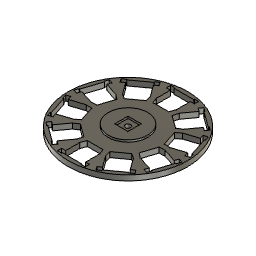
27.10_only_turel_cap (Autodesk Fusion 360 design; units mm, degrees)
Autodesk Fusion 360 part; units mm, degrees
(part 1 of 2)
sketch "Sketch1" plane through (0, 0, 0) normal (0, 0, 1) x (1, 0, 0)
  line L0 (0, -55) -> (0, -85)
  line L1 (0, -85) -> (18.6, -85)
  line L2 (18.6, -85) -> (18.6, -82.7)
  line L3 (18.6, -82.7) -> (13.6, -82.7)
  line L4 (0, -55) -> (5.5, -55)
  line L5 (0, -60) -> (12, -60) construction
  line L6 (5.5, -55) -> (12, -60)
  line L7 (12, -60) -> (13.6, -82.7)
  dimension "d1" = 30
  dimension "d3" = 18.6
  dimension "d4" = 2.3
  dimension "d5" = 5
  dimension "d6" = 5.5
  dimension "d7" = 12
  dimension "d8" = 5
  dimension "d20" = 85
  constraint vertical L0
  constraint coincident origin L0
  constraint perpendicular L0 L1
  constraint perpendicular L1 L2
  constraint perpendicular L2 L3
  constraint perpendicular L0 L4
  constraint coincident L0 L5.start
  constraint perpendicular L0 L5
  measures "d1" distance of L0.start L0.end
  measures "d3" distance of L0.end L1.end
  measures "d4" distance of L1.end L2.end
  measures "d5" distance of L2.end L3.end
  measures "d6" distance of L0.start L4.end
  measures "d7" distance of L5.start L5.end
  measures "d8" distance of L4 L5
  measures "d20" distance of origin L1
revolve "Revolve1" add sketch "Sketch1" angle 360 about axis through (0, -55, 0) along (0, -1, 0) makes body 1
sketch "Sketch2" plane through (0, 0, 0) normal (0, 0, 1) x (1, 0, 0)
  line L0 (-5.5, -55) -> (5.5, -55)
  line L1 (-18.6, -82.7) -> (-13.6, -82.7)
  line L2 (13.6, -82.7) -> (18.6, -82.7)
  line L3 (-18.6, -85) -> (18.6, -85)
  line L4 (-5.5, -55) -> (-12, -60)
  line L5 (5.5, -55) -> (12, -60)
  line L6 (-12, -60) -> (-13.6, -82.7)
  line L7 (12, -60) -> (13.6, -82.7)
  line L8 (-18.6, -82.7) -> (-18.6, -85)
  line L9 (18.6, -82.7) -> (18.6, -85)
  line L10 (0, -85) -> (0, -55) construction
  line L11 (-20.1, -85) -> (20.1, -85)
  line L12 (20.1, -85) -> (20.1, -81)
  line L13 (20.1, -81) -> (15.1, -81)
  line L14 (15.1, -81) -> (15.1, -58.2437)
  line L15 (-12, -60) -> (12, -60) construction
  line L16 (0, -55) -> (0, -50) construction
  line L17 (-12, -50) -> (12, -50)
  line L18 (15.1, -58.2437) -> (12, -50)
  line L19 (-15.1, -58.2437) -> (-12, -50)
  line L20 (-15.1, -81) -> (-15.1, -58.2437)
  line L21 (-20.1, -81) -> (-15.1, -81)
  line L22 (-20.1, -85) -> (-20.1, -81)
  dimension "d10" = 1.5
  dimension "d11" = 4
  dimension "d12" = 5
  dimension "d14" = 5
  constraint midpoint L3 L10.start
  constraint midpoint L0 L10.end
  constraint parallel L3 L11
  constraint midpoint L10.start L11
  constraint perpendicular L11 L12
  constraint perpendicular L12 L13
  constraint perpendicular L13 L14
  constraint equal L7 L14
  constraint coincident L4.end L6.start
  constraint coincident L5.end L7.start
  constraint perpendicular L0 L16
  constraint parallel L15 L17
  constraint midpoint L16.end L17
  constraint equal L15 L17
  constraint symmetric L10 L11.end L11.start
  constraint symmetric L10 L12.end L21.start
  constraint symmetric L10 L13.end L20.start
  constraint symmetric L10 L14.end L19.start
  constraint symmetric L10 L17.end L17.start
  measures "d10" distance of L3.end L11.end
  measures "d11" distance of L11.end L12.end
  measures "d12" distance of L12.end L13.end
  measures "d14" distance of L10.end L16.end
sketch "Sketch3" plane through (0, 0, 0) normal (0, 0, 1) x (1, 0, 0)
  line L0 (-12, -50) -> (12, -50)
  line L1 (15.1, -58.2437) -> (12, -50)
  line L2 (15.1, -81) -> (15.1, -58.2437)
  line L3 (-15.1, -81) -> (-15.1, -58.2437)
  line L4 (-15.1, -58.2437) -> (-12, -50)
  line L5 (20.1, -81) -> (15.1, -81)
  line L6 (-20.1, -85) -> (20.1, -85)
  line L7 (20.1, -85) -> (20.1, -81)
  line L8 (-20.1, -85) -> (-20.1, -81)
  line L9 (-20.1, -81) -> (-15.1, -81)
  circle A0 centre (0, 0) radius 91
  line L10 (-12, -50) -> (12, -50)
  line L11 (15.1, -58.2437) -> (15.1, -81)
  line L12 (20.1, -81) -> (20.1, -85)
  line L13 (20.1, -81) -> (15.1, -81)
  line L14 (15.1, -58.2437) -> (12, -50)
  line L15 (-12, -50) -> (-15.1, -58.2437)
  line L16 (-15.1, -58.2437) -> (-15.1, -81)
  line L17 (-15.1, -81) -> (-20.1, -81)
  line L18 (-20.1, -81) -> (-20.1, -85)
  line L19 (-20.1, -85) -> (20.1, -85)
  line L20 (19.6811, -47.5043) -> (39.0975, -33.3974)
  line L21 (46.4509, -38.2446) -> (39.0975, -33.3974)
  line L22 (46.4509, -38.2446) -> (59.8268, -56.6548)
  line L23 (63.8718, -53.7159) -> (59.8268, -56.6548)
  line L24 (63.8718, -53.7159) -> (66.223, -56.952)
  line L25 (33.7005, -80.5809) -> (66.223, -56.952)
  line L26 (31.3494, -77.3449) -> (33.7005, -80.5809)
  line L27 (35.3944, -74.4059) -> (31.3494, -77.3449)
  line L28 (22.0186, -55.9957) -> (35.3944, -74.4059)
  line L29 (19.6811, -47.5043) -> (22.0186, -55.9957)
  line L30 (43.8446, -26.8635) -> (51.261, -4.0382)
  line L31 (60.0592, -3.6373) -> (51.261, -4.0382)
  line L32 (60.0592, -3.6373) -> (81.7017, -10.6694)
  line L33 (83.2468, -5.9141) -> (81.7017, -10.6694)
  line L34 (83.2468, -5.9141) -> (87.051, -7.1502)
  line L35 (74.6286, -45.3827) -> (87.051, -7.1502)
  line L36 (70.8243, -44.1466) -> (74.6286, -45.3827)
  line L37 (72.3694, -39.3913) -> (70.8243, -44.1466)
  line L38 (50.7269, -32.3592) -> (72.3694, -39.3913)
  line L39 (43.8446, -26.8635) -> (50.7269, -32.3592)
  line L40 (51.261, 4.0382) -> (43.8446, 26.8635)
  line L41 (50.7269, 32.3592) -> (43.8446, 26.8635)
  line L42 (50.7269, 32.3592) -> (72.3694, 39.3913)
  line L43 (70.8243, 44.1466) -> (72.3694, 39.3913)
  line L44 (70.8243, 44.1466) -> (74.6286, 45.3827)
  line L45 (87.051, 7.1502) -> (74.6286, 45.3827)
  line L46 (83.2468, 5.9141) -> (87.051, 7.1502)
  line L47 (81.7017, 10.6694) -> (83.2468, 5.9141)
  line L48 (60.0592, 3.6373) -> (81.7017, 10.6694)
  line L49 (51.261, 4.0382) -> (60.0592, 3.6373)
  line L50 (39.0975, 33.3974) -> (19.6811, 47.5043)
  line L51 (22.0186, 55.9957) -> (19.6811, 47.5043)
  line L52 (22.0186, 55.9957) -> (35.3944, 74.4059)
  line L53 (31.3494, 77.3449) -> (35.3944, 74.4059)
  line L54 (31.3494, 77.3449) -> (33.7005, 80.5809)
  line L55 (66.223, 56.952) -> (33.7005, 80.5809)
  line L56 (63.8718, 53.7159) -> (66.223, 56.952)
  line L57 (59.8268, 56.6548) -> (63.8718, 53.7159)
  line L58 (46.4509, 38.2446) -> (59.8268, 56.6548)
  line L59 (39.0975, 33.3974) -> (46.4509, 38.2446)
  line L60 (12, 50) -> (-12, 50)
  line L61 (-15.1, 58.2437) -> (-12, 50)
  line L62 (-15.1, 58.2437) -> (-15.1, 81)
  line L63 (-20.1, 81) -> (-15.1, 81)
  line L64 (-20.1, 81) -> (-20.1, 85)
  line L65 (20.1, 85) -> (-20.1, 85)
  line L66 (20.1, 81) -> (20.1, 85)
  line L67 (15.1, 81) -> (20.1, 81)
  line L68 (15.1, 58.2437) -> (15.1, 81)
  line L69 (12, 50) -> (15.1, 58.2437)
  line L70 (-19.6811, 47.5043) -> (-39.0975, 33.3974)
  line L71 (-46.4509, 38.2446) -> (-39.0975, 33.3974)
  line L72 (-46.4509, 38.2446) -> (-59.8268, 56.6548)
  line L73 (-63.8718, 53.7159) -> (-59.8268, 56.6548)
  line L74 (-63.8718, 53.7159) -> (-66.223, 56.952)
  line L75 (-33.7005, 80.5809) -> (-66.223, 56.952)
  line L76 (-31.3494, 77.3449) -> (-33.7005, 80.5809)
  line L77 (-35.3944, 74.4059) -> (-31.3494, 77.3449)
  line L78 (-22.0186, 55.9957) -> (-35.3944, 74.4059)
  line L79 (-19.6811, 47.5043) -> (-22.0186, 55.9957)
  line L80 (-43.8446, 26.8635) -> (-51.261, 4.0382)
  line L81 (-60.0592, 3.6373) -> (-51.261, 4.0382)
  line L82 (-60.0592, 3.6373) -> (-81.7017, 10.6694)
  line L83 (-83.2468, 5.9141) -> (-81.7017, 10.6694)
  line L84 (-83.2468, 5.9141) -> (-87.051, 7.1502)
  line L85 (-74.6286, 45.3827) -> (-87.051, 7.1502)
  line L86 (-70.8243, 44.1466) -> (-74.6286, 45.3827)
  line L87 (-72.3694, 39.3913) -> (-70.8243, 44.1466)
  line L88 (-50.7269, 32.3592) -> (-72.3694, 39.3913)
  line L89 (-43.8446, 26.8635) -> (-50.7269, 32.3592)
  line L90 (-51.261, -4.0382) -> (-43.8446, -26.8635)
  line L91 (-50.7269, -32.3592) -> (-43.8446, -26.8635)
  line L92 (-50.7269, -32.3592) -> (-72.3694, -39.3913)
  line L93 (-70.8243, -44.1466) -> (-72.3694, -39.3913)
  line L94 (-70.8243, -44.1466) -> (-74.6286, -45.3827)
  line L95 (-87.051, -7.1502) -> (-74.6286, -45.3827)
  line L96 (-83.2468, -5.9141) -> (-87.051, -7.1502)
  line L97 (-81.7017, -10.6694) -> (-83.2468, -5.9141)
  line L98 (-60.0592, -3.6373) -> (-81.7017, -10.6694)
  line L99 (-51.261, -4.0382) -> (-60.0592, -3.6373)
  line L100 (-39.0975, -33.3974) -> (-19.6811, -47.5043)
  line L101 (-22.0186, -55.9957) -> (-19.6811, -47.5043)
  line L102 (-22.0186, -55.9957) -> (-35.3944, -74.4059)
  line L103 (-31.3494, -77.3449) -> (-35.3944, -74.4059)
  line L104 (-31.3494, -77.3449) -> (-33.7005, -80.5809)
  line L105 (-66.223, -56.952) -> (-33.7005, -80.5809)
  line L106 (-63.8718, -53.7159) -> (-66.223, -56.952)
  line L107 (-59.8268, -56.6548) -> (-63.8718, -53.7159)
  line L108 (-46.4509, -38.2446) -> (-59.8268, -56.6548)
  line L109 (-39.0975, -33.3974) -> (-46.4509, -38.2446)
  circle A1 centre (0, 0) radius 4.05
  dimension "d15" = 182
  dimension "d19" = 360
  dimension "d28" = 8.1
  constraint coincident A0.centre A1.centre
  constraint coincident L0.start L4.end
  constraint coincident L0.end L1.end
  constraint coincident L1.start L2.end
  constraint coincident L2.start L5.end
  constraint coincident L5.start L7.end
  constraint coincident L6.end L7.start
  constraint coincident L3.end L4.start
  constraint coincident L3.start L9.end
  constraint coincident L8.end L9.start
  constraint coincident L6.start L8.start
  measures "d15" diameter of A0
  measures "d28" diameter of A1
extrude "Extrude1" add sketch "Sketch3" along normal blind 8 separate body makes body 2
sketch "Sketch4" plane through (0, 0, 8) normal (0, 0, 1) x (-1, 0, 0)
  line L0 (43.8446, 26.8635) -> (50.7269, 32.3592)
  line L1 (50.7269, 32.3592) -> (72.3694, 39.3913)
  line L2 (72.3694, 39.3913) -> (70.8243, 44.1466)
  line L3 (70.8243, 44.1466) -> (74.6286, 45.3827)
  line L4 (74.6286, 45.3827) -> (87.051, 7.1502)
  line L5 (87.051, 7.1502) -> (83.2468, 5.9141)
  line L6 (83.2468, 5.9141) -> (81.7017, 10.6694)
  line L7 (81.7017, 10.6694) -> (60.0592, 3.6373)
  line L8 (60.0592, 3.6373) -> (51.261, 4.0382)
  line L9 (51.261, 4.0382) -> (43.8446, 26.8635)
  line L10 (19.6811, 47.5043) -> (22.0186, 55.9957)
  line L11 (22.0186, 55.9957) -> (35.3944, 74.4059)
  line L12 (35.3944, 74.4059) -> (31.3494, 77.3449)
  line L13 (31.3494, 77.3449) -> (33.7005, 80.5809)
  line L14 (33.7005, 80.5809) -> (66.223, 56.952)
  line L15 (66.223, 56.952) -> (63.8718, 53.7159)
  line L16 (63.8718, 53.7159) -> (59.8268, 56.6548)
  line L17 (59.8268, 56.6548) -> (46.4509, 38.2446)
  line L18 (46.4509, 38.2446) -> (39.0975, 33.3974)
  line L19 (39.0975, 33.3974) -> (19.6811, 47.5043)
  line L20 (51.261, -4.0382) -> (60.0592, -3.6373)
  line L21 (60.0592, -3.6373) -> (81.7017, -10.6694)
  line L22 (81.7017, -10.6694) -> (83.2468, -5.9141)
  line L23 (83.2468, -5.9141) -> (87.051, -7.1502)
  line L24 (87.051, -7.1502) -> (74.6286, -45.3827)
  line L25 (74.6286, -45.3827) -> (70.8243, -44.1466)
  line L26 (70.8243, -44.1466) -> (72.3694, -39.3913)
  line L27 (72.3694, -39.3913) -> (50.7269, -32.3592)
  line L28 (50.7269, -32.3592) -> (43.8446, -26.8635)
  line L29 (43.8446, -26.8635) -> (51.261, -4.0382)
  line L30 (12, -50) -> (15.1, -58.2437)
  line L31 (15.1, -58.2437) -> (15.1, -81)
  line L32 (15.1, -81) -> (20.1, -81)
  line L33 (20.1, -81) -> (20.1, -85)
  line L34 (20.1, -85) -> (-20.1, -85)
  line L35 (-20.1, -85) -> (-20.1, -81)
  line L36 (-20.1, -81) -> (-15.1, -81)
  line L37 (-15.1, -81) -> (-15.1, -58.2437)
  line L38 (-15.1, -58.2437) -> (-12, -50)
  line L39 (-12, -50) -> (12, -50)
  line L40 (-19.6811, -47.5043) -> (-22.0186, -55.9957)
  line L41 (-22.0186, -55.9957) -> (-35.3944, -74.4059)
  line L42 (-35.3944, -74.4059) -> (-31.3494, -77.3449)
  line L43 (-31.3494, -77.3449) -> (-33.7005, -80.5809)
  line L44 (-33.7005, -80.5809) -> (-66.223, -56.952)
  line L45 (-66.223, -56.952) -> (-63.8718, -53.7159)
  line L46 (-63.8718, -53.7159) -> (-59.8268, -56.6548)
  line L47 (-59.8268, -56.6548) -> (-46.4509, -38.2446)
  line L48 (-46.4509, -38.2446) -> (-39.0975, -33.3974)
  line L49 (-39.0975, -33.3974) -> (-19.6811, -47.5043)
  line L50 (-51.261, 4.0382) -> (-60.0592, 3.6373)
  line L51 (-60.0592, 3.6373) -> (-81.7017, 10.6694)
  line L52 (-81.7017, 10.6694) -> (-83.2468, 5.9141)
  line L53 (-83.2468, 5.9141) -> (-87.051, 7.1502)
  line L54 (-87.051, 7.1502) -> (-74.6286, 45.3827)
  line L55 (-74.6286, 45.3827) -> (-70.8243, 44.1466)
  line L56 (-70.8243, 44.1466) -> (-72.3694, 39.3913)
  line L57 (-72.3694, 39.3913) -> (-50.7269, 32.3592)
  line L58 (-50.7269, 32.3592) -> (-43.8446, 26.8635)
  line L59 (-43.8446, 26.8635) -> (-51.261, 4.0382)
  line L60 (15.1, 58.2437) -> (12, 50)
  line L61 (12, 50) -> (-12, 50)
  line L62 (-12, 50) -> (-15.1, 58.2437)
  line L63 (-15.1, 58.2437) -> (-15.1, 81)
  line L64 (-15.1, 81) -> (-20.1, 81)
  line L65 (-20.1, 81) -> (-20.1, 85)
  line L66 (-20.1, 85) -> (20.1, 85)
  line L67 (20.1, 85) -> (20.1, 81)
  line L68 (20.1, 81) -> (15.1, 81)
  line L69 (15.1, 81) -> (15.1, 58.2437)
  line L70 (-39.0975, 33.3974) -> (-46.4509, 38.2446)
  line L71 (-46.4509, 38.2446) -> (-59.8268, 56.6548)
  line L72 (-59.8268, 56.6548) -> (-63.8718, 53.7159)
  line L73 (-63.8718, 53.7159) -> (-66.223, 56.952)
  line L74 (-66.223, 56.952) -> (-33.7005, 80.5809)
  line L75 (-33.7005, 80.5809) -> (-31.3494, 77.3449)
  line L76 (-31.3494, 77.3449) -> (-35.3944, 74.4059)
  line L77 (-35.3944, 74.4059) -> (-22.0186, 55.9957)
  line L78 (-22.0186, 55.9957) -> (-19.6811, 47.5043)
  line L79 (-19.6811, 47.5043) -> (-39.0975, 33.3974)
  line L80 (39.0975, -33.3974) -> (46.4509, -38.2446)
  line L81 (46.4509, -38.2446) -> (59.8268, -56.6548)
  line L82 (59.8268, -56.6548) -> (63.8718, -53.7159)
  line L83 (63.8718, -53.7159) -> (66.223, -56.952)
  line L84 (66.223, -56.952) -> (33.7005, -80.5809)
  line L85 (33.7005, -80.5809) -> (31.3494, -77.3449)
  line L86 (31.3494, -77.3449) -> (35.3944, -74.4059)
  line L87 (35.3944, -74.4059) -> (22.0186, -55.9957)
  line L88 (22.0186, -55.9957) -> (19.6811, -47.5043)
  line L89 (19.6811, -47.5043) -> (39.0975, -33.3974)
  line L90 (-43.8446, -26.8635) -> (-50.7269, -32.3592)
  line L91 (-50.7269, -32.3592) -> (-72.3694, -39.3913)
  line L92 (-72.3694, -39.3913) -> (-70.8243, -44.1466)
  line L93 (-70.8243, -44.1466) -> (-74.6286, -45.3827)
  line L94 (-74.6286, -45.3827) -> (-87.051, -7.1502)
  line L95 (-87.051, -7.1502) -> (-83.2468, -5.9141)
  line L96 (-83.2468, -5.9141) -> (-81.7017, -10.6694)
  line L97 (-81.7017, -10.6694) -> (-60.0592, -3.6373)
  line L98 (-60.0592, -3.6373) -> (-51.261, -4.0382)
  line L99 (-51.261, -4.0382) -> (-43.8446, -26.8635)
  circle A0 centre (0, 0) radius 91
  line L100 (-20.1, 81) -> (-15.1, 81)
  line L101 (-20.1, 81) -> (-20.1, 85)
  line L102 (20.1, 85) -> (-20.1, 85)
  line L103 (20.1, 81) -> (20.1, 85)
  line L104 (15.1, 81) -> (20.1, 81)
  line L105 (-15.1, 81) -> (-20.1, 81)
  line L106 (-20.1, 85) -> (-20.1, 81)
  line L107 (-20.1, 85) -> (-14.95, 85)
  line L108 (-14.95, 85) -> (-14.95, 86.15)
  line L109 (-15.1, 81) -> (-15.1, 79.85)
  line L110 (-15.1, 79.85) -> (-21.25, 79.85)
  line L111 (-21.25, 79.85) -> (-21.25, 86.15)
  line L112 (-21.25, 86.15) -> (-14.95, 86.15)
  line L113 (0, 0) -> (0, 91) construction
  line L114 (15.1, 81) -> (15.1, 79.85)
  line L115 (15.1, 79.85) -> (21.25, 79.85)
  line L116 (21.25, 79.85) -> (21.25, 86.15)
  line L117 (21.25, 86.15) -> (14.95, 86.15)
  line L118 (14.95, 85) -> (14.95, 86.15)
  line L119 (20.1, 85) -> (14.95, 85)
  line L120 (20.1, 85) -> (20.1, 81)
  line L121 (15.1, 81) -> (20.1, 81)
  circle A1 centre (0, 0) radius 4.05
  dimension "d21" = 5.15
  dimension "d22" = 6.3
  dimension "d23" = 6.3
  constraint coincident L63.end L64.start
  constraint coincident L64.end L65.start
  constraint coincident L65.end L66.start
  constraint coincident L66 L107.end
  constraint perpendicular L65 L107
  constraint perpendicular L102 L108
  constraint coincident L63 L109.end
  constraint perpendicular L64 L109
  constraint perpendicular L63 L110
  constraint perpendicular L110 L111
  constraint perpendicular L108 L112
  constraint equal L108 L109
  constraint coincident A0.centre L113.start
  constraint coincident A0 L113.end
  constraint perpendicular L102 L113
  constraint symmetric L63.end L113 L68.end
  constraint symmetric L64.end L113 L67.end
  constraint symmetric L65.end L113 L66.end
  constraint symmetric L107.end L113 L118.start
  constraint symmetric L108.end L113 L117.end
  constraint symmetric L109.end L113 L114.end
  constraint symmetric L110.end L113 L115.end
  constraint symmetric L111.end L113 L116.end
  measures "d21" distance of L65.end L107.end
  measures "d22" distance of L108.end L111.end
  measures "d23" distance of L110.end L111.end
extrude "Extrude2" cut sketch "Sketch4" against normal blind 25 contours L66 L67 L68 L69 L102 L103 L104 L114 L115 L116 L117 L118 L119 L120 L121 | L63 L64 L65 L66 L100 L101 L102 L105 L106 L107 L108 L109 L110 L111 L112 bodies 2
pattern_circular "C-Pattern1" count 10 over 360 about axis through (0, 0, 1.75) along (0, 0, 1) of "Extrude2"
sketch "Sketch5" plane through (0, 0, 0) normal (0, 1, 0) x (1, 0, 0)
  line L0 (0, 0) -> (0, -592)
  dimension "d31" = 592
  constraint coincident L0.start origin
  constraint vertical L0
  measures "d31" distance of L0.start L0.end
ref_plane "WorkPlane1" through (0, 0, 296) normal (0, 0, 1) x (1, 0, 0)
sketch "Sketch6" plane through (0, 0, 8) normal (0, 0, 1) x (-1, 0, 0)
  line L0 (14.95, 85) -> (14.95, 86.15)
  line L1 (14.95, 86.15) -> (21.25, 86.15)
  line L2 (21.25, 86.15) -> (21.25, 79.85)
  line L3 (21.25, 79.85) -> (15.1, 79.85)
  line L4 (15.1, 79.85) -> (15.1, 58.2437)
  line L5 (15.1, 58.2437) -> (12, 50)
  line L6 (12, 50) -> (-12, 50)
  line L7 (-12, 50) -> (-15.1, 58.2437)
  line L8 (-15.1, 58.2437) -> (-15.1, 79.85)
  line L9 (-15.1, 79.85) -> (-21.25, 79.85)
  line L10 (-21.25, 79.85) -> (-21.25, 86.15)
  line L11 (-21.25, 86.15) -> (-14.95, 86.15)
  line L12 (-14.95, 86.15) -> (-14.95, 85)
  line L13 (-14.95, 85) -> (14.95, 85)
  circle A0 centre (0, 0) radius 4.05
  line L14 (85.4596, 12.0481) -> (86.5533, 12.4035)
  line L15 (86.5533, 12.4035) -> (88.5001, 6.4119)
  line L16 (88.5001, 6.4119) -> (82.5085, 4.4651)
  line L17 (82.5085, 4.4651) -> (80.608, 10.3141)
  line L18 (80.608, 10.3141) -> (60.0592, 3.6373)
  line L19 (60.0592, 3.6373) -> (51.261, 4.0382)
  line L20 (51.261, 4.0382) -> (43.8446, 26.8635)
  line L21 (43.8446, 26.8635) -> (50.7269, 32.3592)
  line L22 (50.7269, 32.3592) -> (71.2757, 39.036)
  line L23 (71.2757, 39.036) -> (69.3753, 44.885)
  line L24 (69.3753, 44.885) -> (75.3669, 46.8318)
  line L25 (75.3669, 46.8318) -> (77.3137, 40.8401)
  line L26 (77.3137, 40.8401) -> (76.22, 40.4847)
  line L27 (76.22, 40.4847) -> (85.4596, 12.0481)
  line L28 (62.0566, 59.9791) -> (62.7325, 60.9094)
  line L29 (62.7325, 60.9094) -> (67.8293, 57.2064)
  line L30 (67.8293, 57.2064) -> (64.1263, 52.1096)
  line L31 (64.1263, 52.1096) -> (59.1508, 55.7244)
  line L32 (59.1508, 55.7244) -> (46.4509, 38.2446)
  line L33 (46.4509, 38.2446) -> (39.0975, 33.3974)
  line L34 (39.0975, 33.3974) -> (19.6811, 47.5043)
  line L35 (19.6811, 47.5043) -> (22.0186, 55.9957)
  line L36 (22.0186, 55.9957) -> (34.7185, 73.4756)
  line L37 (34.7185, 73.4756) -> (29.743, 77.0904)
  line L38 (29.743, 77.0904) -> (33.4461, 82.1873)
  line L39 (33.4461, 82.1873) -> (38.5429, 78.4842)
  line L40 (38.5429, 78.4842) -> (37.8669, 77.5538)
  line L41 (37.8669, 77.5538) -> (62.0566, 59.9791)
  line L42 (-14.95, -85) -> (-14.95, -86.15)
  line L43 (-14.95, -86.15) -> (-21.25, -86.15)
  line L44 (-21.25, -86.15) -> (-21.25, -79.85)
  line L45 (-21.25, -79.85) -> (-15.1, -79.85)
  line L46 (-15.1, -79.85) -> (-15.1, -58.2437)
  line L47 (-15.1, -58.2437) -> (-12, -50)
  line L48 (-12, -50) -> (12, -50)
  line L49 (12, -50) -> (15.1, -58.2437)
  line L50 (15.1, -58.2437) -> (15.1, -79.85)
  line L51 (15.1, -79.85) -> (21.25, -79.85)
  line L52 (21.25, -79.85) -> (21.25, -86.15)
  line L53 (21.25, -86.15) -> (14.95, -86.15)
  line L54 (14.95, -86.15) -> (14.95, -85)
  line L55 (14.95, -85) -> (-14.95, -85)
  line L56 (37.8669, -77.5538) -> (38.5429, -78.4842)
  line L57 (38.5429, -78.4842) -> (33.4461, -82.1873)
  line L58 (33.4461, -82.1873) -> (29.743, -77.0904)
  line L59 (29.743, -77.0904) -> (34.7185, -73.4756)
  line L60 (34.7185, -73.4756) -> (22.0186, -55.9957)
  line L61 (22.0186, -55.9957) -> (19.6811, -47.5043)
  line L62 (19.6811, -47.5043) -> (39.0975, -33.3974)
  line L63 (39.0975, -33.3974) -> (46.4509, -38.2446)
  line L64 (46.4509, -38.2446) -> (59.1508, -55.7244)
  line L65 (59.1508, -55.7244) -> (64.1263, -52.1096)
  line L66 (64.1263, -52.1096) -> (67.8293, -57.2064)
  line L67 (67.8293, -57.2064) -> (62.7325, -60.9094)
  line L68 (62.7325, -60.9094) -> (62.0566, -59.9791)
  line L69 (62.0566, -59.9791) -> (37.8669, -77.5538)
  line L70 (-85.4596, -12.0481) -> (-86.5533, -12.4035)
  line L71 (-86.5533, -12.4035) -> (-88.5001, -6.4119)
  line L72 (-88.5001, -6.4119) -> (-82.5085, -4.4651)
  line L73 (-82.5085, -4.4651) -> (-80.608, -10.3141)
  line L74 (-80.608, -10.3141) -> (-60.0592, -3.6373)
  line L75 (-60.0592, -3.6373) -> (-51.261, -4.0382)
  line L76 (-51.261, -4.0382) -> (-43.8446, -26.8635)
  line L77 (-43.8446, -26.8635) -> (-50.7269, -32.3592)
  line L78 (-50.7269, -32.3592) -> (-71.2757, -39.036)
  line L79 (-71.2757, -39.036) -> (-69.3753, -44.885)
  line L80 (-69.3753, -44.885) -> (-75.3669, -46.8318)
  line L81 (-75.3669, -46.8318) -> (-77.3137, -40.8401)
  line L82 (-77.3137, -40.8401) -> (-76.22, -40.4847)
  line L83 (-76.22, -40.4847) -> (-85.4596, -12.0481)
  line L84 (-76.22, 40.4847) -> (-77.3137, 40.8401)
  line L85 (-77.3137, 40.8401) -> (-75.3669, 46.8318)
  line L86 (-75.3669, 46.8318) -> (-69.3753, 44.885)
  line L87 (-69.3753, 44.885) -> (-71.2757, 39.036)
  line L88 (-71.2757, 39.036) -> (-50.7269, 32.3592)
  line L89 (-50.7269, 32.3592) -> (-43.8446, 26.8635)
  line L90 (-43.8446, 26.8635) -> (-51.261, 4.0382)
  line L91 (-51.261, 4.0382) -> (-60.0592, 3.6373)
  line L92 (-60.0592, 3.6373) -> (-80.608, 10.3141)
  line L93 (-80.608, 10.3141) -> (-82.5085, 4.4651)
  line L94 (-82.5085, 4.4651) -> (-88.5001, 6.4119)
  line L95 (-88.5001, 6.4119) -> (-86.5533, 12.4035)
  line L96 (-86.5533, 12.4035) -> (-85.4596, 12.0481)
  line L97 (-85.4596, 12.0481) -> (-76.22, 40.4847)
  line L98 (-62.0566, -59.9791) -> (-62.7325, -60.9094)
  line L99 (-62.7325, -60.9094) -> (-67.8293, -57.2064)
  line L100 (-67.8293, -57.2064) -> (-64.1263, -52.1096)
  line L101 (-64.1263, -52.1096) -> (-59.1508, -55.7244)
  line L102 (-59.1508, -55.7244) -> (-46.4509, -38.2446)
  line L103 (-46.4509, -38.2446) -> (-39.0975, -33.3974)
  line L104 (-39.0975, -33.3974) -> (-19.6811, -47.5043)
  line L105 (-19.6811, -47.5043) -> (-22.0186, -55.9957)
  line L106 (-22.0186, -55.9957) -> (-34.7185, -73.4756)
  line L107 (-34.7185, -73.4756) -> (-29.743, -77.0904)
  line L108 (-29.743, -77.0904) -> (-33.4461, -82.1873)
  line L109 (-33.4461, -82.1873) -> (-38.5429, -78.4842)
  line L110 (-38.5429, -78.4842) -> (-37.8669, -77.5538)
  line L111 (-37.8669, -77.5538) -> (-62.0566, -59.9791)
  line L112 (76.22, -40.4847) -> (77.3137, -40.8401)
  line L113 (77.3137, -40.8401) -> (75.3669, -46.8318)
  line L114 (75.3669, -46.8318) -> (69.3753, -44.885)
  line L115 (69.3753, -44.885) -> (71.2757, -39.036)
  line L116 (71.2757, -39.036) -> (50.7269, -32.3592)
  line L117 (50.7269, -32.3592) -> (43.8446, -26.8635)
  line L118 (43.8446, -26.8635) -> (51.261, -4.0382)
  line L119 (51.261, -4.0382) -> (60.0592, -3.6373)
  line L120 (60.0592, -3.6373) -> (80.608, -10.3141)
  line L121 (80.608, -10.3141) -> (82.5085, -4.4651)
  line L122 (82.5085, -4.4651) -> (88.5001, -6.4119)
  line L123 (88.5001, -6.4119) -> (86.5533, -12.4035)
  line L124 (86.5533, -12.4035) -> (85.4596, -12.0481)
  line L125 (85.4596, -12.0481) -> (76.22, -40.4847)
  line L126 (-37.8669, 77.5538) -> (-38.5429, 78.4842)
  line L127 (-38.5429, 78.4842) -> (-33.4461, 82.1873)
  line L128 (-33.4461, 82.1873) -> (-29.743, 77.0904)
  line L129 (-29.743, 77.0904) -> (-34.7185, 73.4756)
  line L130 (-34.7185, 73.4756) -> (-22.0186, 55.9957)
  line L131 (-22.0186, 55.9957) -> (-19.6811, 47.5043)
  line L132 (-19.6811, 47.5043) -> (-39.0975, 33.3974)
  line L133 (-39.0975, 33.3974) -> (-46.4509, 38.2446)
  line L134 (-46.4509, 38.2446) -> (-59.1508, 55.7244)
  line L135 (-59.1508, 55.7244) -> (-64.1263, 52.1096)
  line L136 (-64.1263, 52.1096) -> (-67.8293, 57.2064)
  line L137 (-67.8293, 57.2064) -> (-62.7325, 60.9094)
  line L138 (-62.7325, 60.9094) -> (-62.0566, 59.9791)
  line L139 (-62.0566, 59.9791) -> (-37.8669, 77.5538)
  circle A1 centre (0, 0) radius 91
  line L140 (10.075, -10.075) -> (-10.075, -10.075)
  line L141 (-10.075, -10.075) -> (-10.075, 10.075)
  line L142 (-10.075, 10.075) -> (10.075, 10.075)
  line L143 (10.075, 10.075) -> (10.075, -10.075)
  line L144 (10.075, -10.075) -> (-10.075, 10.075) construction
  circle A2 centre (0, 0) radius 30
  line L145 (20.1, 85) -> (-20.1, 85)
  line L146 (-20.1, 81) -> (-20.1, 85)
  line L147 (-20.1, 81) -> (-15.1, 81)
  line L148 (-15.1, 58.2437) -> (-15.1, 81)
  line L149 (15.1, 58.2437) -> (15.1, 81)
  line L150 (15.1, 81) -> (20.1, 81)
  line L151 (20.1, 81) -> (20.1, 85)
  line L152 (10.3486, 85) -> (-10.3486, 85)
  arc A3 (10.3486, 85) -> (-15.1, 81) centre (0, 67.8855) ccw
  line L153 (-41.5895, 74.8492) -> (-58.334, 62.6837)
  arc A4 (-41.5895, 74.8492) -> (-59.8268, 56.6548) centre (-39.9021, 54.9205) ccw
  line L154 (-77.6419, 36.1086) -> (-84.0377, 16.4243)
  arc A5 (-77.6419, 36.1086) -> (-81.7017, 10.6694) centre (-64.563, 20.9778) ccw
  line L155 (-84.0377, -16.4243) -> (-77.6419, -36.1086)
  arc A6 (-84.0377, -16.4243) -> (-72.3694, -39.3913) centre (-64.563, -20.9778) ccw
  line L156 (-58.334, -62.6837) -> (-41.5895, -74.8492)
  arc A7 (-58.334, -62.6837) -> (-35.3944, -74.4059) centre (-39.9021, -54.9205) ccw
  line L157 (-10.3486, -85) -> (10.3486, -85)
  arc A8 (-10.3486, -85) -> (15.1, -81) centre (0, -67.8855) ccw
  line L158 (41.5895, -74.8492) -> (58.334, -62.6837)
  arc A9 (41.5895, -74.8492) -> (59.8268, -56.6548) centre (39.9021, -54.9205) ccw
  line L159 (77.6419, -36.1086) -> (84.0377, -16.4243)
  arc A10 (77.6419, -36.1086) -> (81.7017, -10.6694) centre (64.563, -20.9778) ccw
  line L160 (84.0377, 16.4243) -> (77.6419, 36.1086)
  arc A11 (84.0377, 16.4243) -> (72.3694, 39.3913) centre (64.563, 20.9778) ccw
  line L161 (58.334, 62.6837) -> (41.5895, 74.8492)
  arc A12 (58.334, 62.6837) -> (35.3944, 74.4059) centre (39.9021, 54.9205) ccw
  arc A13 (-29.743, -77.0904) -> (-21.25, -79.85) centre (-19.1862, -59.0492) ccw
  line L162 (0, 0) -> (-1.4578, -3.7785)
  line L163 (-10.7987, -27.9891) -> (-29.743, -77.0904)
  line L164 (0, 0) -> (-1.0416, -3.9138)
  line L165 (-7.7152, -28.991) -> (-21.25, -79.85)
  line L166 (7.7152, -28.991) -> (21.25, -79.85)
  arc A14 (21.25, -79.85) -> (29.743, -77.0904) centre (19.1862, -59.0492) ccw
  line L167 (10.7987, -27.9891) -> (29.743, -77.0904)
  line L168 (23.2822, -18.9193) -> (64.1263, -52.1096)
  arc A15 (64.1263, -52.1096) -> (69.3753, -44.885) centre (50.2302, -36.4944) ccw
  line L169 (25.1879, -16.2963) -> (69.3753, -44.885)
  line L170 (29.9562, -1.6211) -> (82.5085, -4.4651)
  arc A16 (82.5085, -4.4651) -> (82.5085, 4.4651) centre (62.088, 0) ccw
  line L171 (29.9562, 1.6211) -> (82.5085, 4.4651)
  line L172 (25.1879, 16.2963) -> (69.3753, 44.885)
  arc A17 (69.3753, 44.885) -> (64.1263, 52.1096) centre (50.2302, 36.4944) ccw
  line L173 (23.2822, 18.9193) -> (64.1263, 52.1096)
  line L174 (10.7987, 27.9891) -> (29.743, 77.0904)
  arc A18 (29.743, 77.0904) -> (21.25, 79.85) centre (19.1862, 59.0492) ccw
  line L175 (7.7152, 28.991) -> (21.25, 79.85)
  line L176 (-7.7152, 28.991) -> (-21.25, 79.85)
  arc A19 (-21.25, 79.85) -> (-29.743, 77.0904) centre (-19.1862, 59.0492) ccw
  line L177 (-10.7987, 27.9891) -> (-29.743, 77.0904)
  line L178 (-23.2822, 18.9193) -> (-64.1263, 52.1096)
  arc A20 (-64.1263, 52.1096) -> (-69.3753, 44.885) centre (-50.2302, 36.4944) ccw
  line L179 (-25.1879, 16.2963) -> (-69.3753, 44.885)
  line L180 (-29.9562, 1.6211) -> (-82.5085, 4.4651)
  arc A21 (-82.5085, 4.4651) -> (-82.5085, -4.4651) centre (-62.088, 0) ccw
  line L181 (-29.9562, -1.6211) -> (-82.5085, -4.4651)
  line L182 (-25.1879, -16.2963) -> (-69.3753, -44.885)
  arc A22 (-69.3753, -44.885) -> (-64.1263, -52.1096) centre (-50.2302, -36.4944) ccw
  line L183 (-23.2822, -18.9193) -> (-64.1263, -52.1096)
  line L184 (0, 0) -> (0, 91) construction
  dimension "d35" = 20.15
  dimension "d36" = 60
  dimension "d44" = 40
  dimension "d47" = 360
  dimension "d93" = 62.088
  dimension "d95" = 360
  constraint horizontal L140
  constraint vertical L141
  constraint horizontal L142
  constraint vertical L143
  constraint equal L140 L141
  constraint midpoint A0.centre L144
  constraint coincident A0.centre A1.centre
  constraint coincident L13 L152.start
  constraint coincident L145 L152.end
  constraint coincident L152.end A3
  constraint coincident L107.end L108.start
  constraint coincident L44.end L45.start
  constraint coincident A2 L163.start
  constraint collinear L162 L163
  constraint coincident A2 L165.start
  constraint collinear L164 L165
  constraint coincident A0 L162.end
  constraint coincident A0 L164.end
  constraint coincident A1 L184.end
  constraint perpendicular L145 L184
  constraint coincident L149.end A3
  measures "d35" distance of L140.start L140.end
  measures "d36" diameter of A2
  measures "d44" diameter of A3
  measures "d93" distance of A0.centre A13.centre
extrude "Extrude3" add sketch "Sketch6" along normal blind 3 contours A2 bodies 2
extrude "Extrude4" [rolled back] along distance -1 taper angle 0
sketch "Sketch7" plane through (0, 0, 0) normal (0, 0, -1) x (1, 0, 0)
  circle A0 centre (0, 0) radius 4.05
  line L0 (-50.7269, 32.3592) -> (-43.8446, 26.8635)
  line L1 (-43.8446, 26.8635) -> (-51.261, 4.0382)
  line L2 (-51.261, 4.0382) -> (-60.0592, 3.6373)
  line L3 (-60.0592, 3.6373) -> (-81.7017, 10.6694)
  line L4 (-81.7017, 10.6694) -> (-83.2468, 5.9141)
  line L5 (-83.2468, 5.9141) -> (-87.051, 7.1502)
  line L6 (-87.051, 7.1502) -> (-74.6286, 45.3827)
  line L7 (-74.6286, 45.3827) -> (-70.8243, 44.1466)
  line L8 (-70.8243, 44.1466) -> (-72.3694, 39.3913)
  line L9 (-72.3694, 39.3913) -> (-50.7269, 32.3592)
  line L10 (-22.0186, 55.9957) -> (-19.6811, 47.5043)
  line L11 (-19.6811, 47.5043) -> (-39.0975, 33.3974)
  line L12 (-39.0975, 33.3974) -> (-46.4509, 38.2446)
  line L13 (-46.4509, 38.2446) -> (-59.8268, 56.6548)
  line L14 (-59.8268, 56.6548) -> (-63.8718, 53.7159)
  line L15 (-63.8718, 53.7159) -> (-66.223, 56.952)
  line L16 (-66.223, 56.952) -> (-33.7005, 80.5809)
  line L17 (-33.7005, 80.5809) -> (-31.3494, 77.3449)
  line L18 (-31.3494, 77.3449) -> (-35.3944, 74.4059)
  line L19 (-35.3944, 74.4059) -> (-22.0186, 55.9957)
  line L20 (-15.1, -58.2437) -> (-12, -50)
  line L21 (-12, -50) -> (12, -50)
  line L22 (12, -50) -> (15.1, -58.2437)
  line L23 (15.1, -58.2437) -> (15.1, -81)
  line L24 (15.1, -81) -> (20.1, -81)
  line L25 (20.1, -81) -> (20.1, -85)
  line L26 (20.1, -85) -> (-20.1, -85)
  line L27 (-20.1, -85) -> (-20.1, -81)
  line L28 (-20.1, -81) -> (-15.1, -81)
  line L29 (-15.1, -81) -> (-15.1, -58.2437)
  line L30 (-46.4509, -38.2446) -> (-39.0975, -33.3974)
  line L31 (-39.0975, -33.3974) -> (-19.6811, -47.5043)
  line L32 (-19.6811, -47.5043) -> (-22.0186, -55.9957)
  line L33 (-22.0186, -55.9957) -> (-35.3944, -74.4059)
  line L34 (-35.3944, -74.4059) -> (-31.3494, -77.3449)
  line L35 (-31.3494, -77.3449) -> (-33.7005, -80.5809)
  line L36 (-33.7005, -80.5809) -> (-66.223, -56.952)
  line L37 (-66.223, -56.952) -> (-63.8718, -53.7159)
  line L38 (-63.8718, -53.7159) -> (-59.8268, -56.6548)
  line L39 (-59.8268, -56.6548) -> (-46.4509, -38.2446)
  line L40 (50.7269, -32.3592) -> (43.8446, -26.8635)
  line L41 (43.8446, -26.8635) -> (51.261, -4.0382)
  line L42 (51.261, -4.0382) -> (60.0592, -3.6373)
  line L43 (60.0592, -3.6373) -> (81.7017, -10.6694)
  line L44 (81.7017, -10.6694) -> (83.2468, -5.9141)
  line L45 (83.2468, -5.9141) -> (87.051, -7.1502)
  line L46 (87.051, -7.1502) -> (74.6286, -45.3827)
  line L47 (74.6286, -45.3827) -> (70.8243, -44.1466)
  line L48 (70.8243, -44.1466) -> (72.3694, -39.3913)
  line L49 (72.3694, -39.3913) -> (50.7269, -32.3592)
  line L50 (60.0592, 3.6373) -> (51.261, 4.0382)
  line L51 (51.261, 4.0382) -> (43.8446, 26.8635)
  line L52 (43.8446, 26.8635) -> (50.7269, 32.3592)
  line L53 (50.7269, 32.3592) -> (72.3694, 39.3913)
  line L54 (72.3694, 39.3913) -> (70.8243, 44.1466)
  line L55 (70.8243, 44.1466) -> (74.6286, 45.3827)
  line L56 (74.6286, 45.3827) -> (87.051, 7.1502)
  line L57 (87.051, 7.1502) -> (83.2468, 5.9141)
  line L58 (83.2468, 5.9141) -> (81.7017, 10.6694)
  line L59 (81.7017, 10.6694) -> (60.0592, 3.6373)
  line L60 (22.0186, -55.9957) -> (19.6811, -47.5043)
  line L61 (19.6811, -47.5043) -> (39.0975, -33.3974)
  line L62 (39.0975, -33.3974) -> (46.4509, -38.2446)
  line L63 (46.4509, -38.2446) -> (59.8268, -56.6548)
  line L64 (59.8268, -56.6548) -> (63.8718, -53.7159)
  line L65 (63.8718, -53.7159) -> (66.223, -56.952)
  line L66 (66.223, -56.952) -> (33.7005, -80.5809)
  line L67 (33.7005, -80.5809) -> (31.3494, -77.3449)
  line L68 (31.3494, -77.3449) -> (35.3944, -74.4059)
  line L69 (35.3944, -74.4059) -> (22.0186, -55.9957)
  line L70 (-12, 50) -> (-15.1, 58.2437)
  line L71 (-15.1, 58.2437) -> (-15.1, 81)
  line L72 (-15.1, 81) -> (-20.1, 81)
  line L73 (-20.1, 81) -> (-20.1, 85)
  line L74 (-20.1, 85) -> (20.1, 85)
  line L75 (20.1, 85) -> (20.1, 81)
  line L76 (20.1, 81) -> (15.1, 81)
  line L77 (15.1, 81) -> (15.1, 58.2437)
  line L78 (15.1, 58.2437) -> (12, 50)
  line L79 (12, 50) -> (-12, 50)
  line L80 (-60.0592, -3.6373) -> (-51.261, -4.0382)
  line L81 (-51.261, -4.0382) -> (-43.8446, -26.8635)
  line L82 (-43.8446, -26.8635) -> (-50.7269, -32.3592)
  line L83 (-50.7269, -32.3592) -> (-72.3694, -39.3913)
  line L84 (-72.3694, -39.3913) -> (-70.8243, -44.1466)
  line L85 (-70.8243, -44.1466) -> (-74.6286, -45.3827)
  line L86 (-74.6286, -45.3827) -> (-87.051, -7.1502)
  line L87 (-87.051, -7.1502) -> (-83.2468, -5.9141)
  line L88 (-83.2468, -5.9141) -> (-81.7017, -10.6694)
  line L89 (-81.7017, -10.6694) -> (-60.0592, -3.6373)
  line L90 (46.4509, 38.2446) -> (39.0975, 33.3974)
  line L91 (39.0975, 33.3974) -> (19.6811, 47.5043)
  line L92 (19.6811, 47.5043) -> (22.0186, 55.9957)
  line L93 (22.0186, 55.9957) -> (35.3944, 74.4059)
  line L94 (35.3944, 74.4059) -> (31.3494, 77.3449)
  line L95 (31.3494, 77.3449) -> (33.7005, 80.5809)
  line L96 (33.7005, 80.5809) -> (66.223, 56.952)
  line L97 (66.223, 56.952) -> (63.8718, 53.7159)
  line L98 (63.8718, 53.7159) -> (59.8268, 56.6548)
  line L99 (59.8268, 56.6548) -> (46.4509, 38.2446)
  circle A1 centre (0, 0) radius 91
  circle A2 centre (0, 0) radius 26.55
  line L100 (-15.1, 58.2437) -> (-15.1, 81)
  line L101 (-12, 50) -> (-15.1, 58.2437)
  line L102 (-12, 50) -> (12, 50)
  line L103 (15.1, 58.2437) -> (12, 50)
  line L104 (15.1, 58.2437) -> (15.1, 81)
  line L105 (20.1, 81) -> (15.1, 81)
  line L106 (20.1, 81) -> (20.1, 85)
  line L107 (-20.1, 85) -> (20.1, 85)
  line L108 (-20.1, 81) -> (-20.1, 85)
  line L109 (-15.1, 81) -> (-20.1, 81)
  arc A3 (15.1, 81) -> (-10.3486, 85) centre (0, 67.8855) ccw
  dimension "d41" = 53.1
  constraint concentric A0 A2
  measures "d41" diameter of A2
extrude "Extrude5" [rolled back] along distance -3.5 taper angle 0
extrude "Extrude6" [rolled back] taper angle 0
ref_plane "WorkPlane6" through (0, 0, -10) normal (0, 0, 1) x (1, 0, 0)
sketch "Sketch10" plane through (0, 0, -10) normal (0, 0, 1) x (1, 0, 0)
  arc A0 (41.5895, -74.8492) -> (58.334, -62.6837) centre (39.9021, -54.9205) ccw
  arc A1 (58.334, 62.6837) -> (41.5895, 74.8492) centre (39.9021, 54.9205) ccw
  arc A2 (-77.6419, 36.1086) -> (-84.0377, 16.4243) centre (-64.563, 20.9778) ccw
  arc A3 (10.3486, 85) -> (-10.3486, 85) centre (0, 67.8855) ccw
  arc A4 (-10.3486, -85) -> (10.3486, -85) centre (0, -67.8855) ccw
  arc A5 (77.6419, -36.1086) -> (84.0377, -16.4243) centre (64.563, -20.9778) ccw
  arc A6 (-41.5895, 74.8492) -> (-58.334, 62.6837) centre (-39.9021, 54.9205) ccw
  arc A7 (-84.0377, -16.4243) -> (-77.6419, -36.1086) centre (-64.563, -20.9778) ccw
  arc A8 (84.0377, 16.4243) -> (77.6419, 36.1086) centre (64.563, 20.9778) ccw
  arc A9 (-58.334, -62.6837) -> (-41.5895, -74.8492) centre (-39.9021, -54.9205) ccw
  line L0 (66.223, -56.952) -> (58.334, -62.6837)
  line L1 (33.7005, 80.5809) -> (41.5895, 74.8492)
  line L2 (-87.051, 7.1502) -> (-84.0377, 16.4243)
  line L3 (-20.1, 85) -> (-10.3486, 85)
  line L4 (20.1, -85) -> (10.3486, -85)
  line L5 (87.051, -7.1502) -> (84.0377, -16.4243)
  line L6 (-66.223, 56.952) -> (-58.334, 62.6837)
  line L7 (-74.6286, -45.3827) -> (-77.6419, -36.1086)
  line L8 (74.6286, 45.3827) -> (77.6419, 36.1086)
  line L9 (-70.8243, -44.1466) -> (-74.6286, -45.3827)
  line L10 (-72.3694, -39.3913) -> (-70.8243, -44.1466)
  line L11 (-50.7269, -32.3592) -> (-72.3694, -39.3913)
  line L12 (-43.8446, -26.8635) -> (-50.7269, -32.3592)
  line L13 (-51.261, -4.0382) -> (-43.8446, -26.8635)
  line L14 (-60.0592, -3.6373) -> (-51.261, -4.0382)
  line L15 (-81.7017, -10.6694) -> (-60.0592, -3.6373)
  line L16 (-83.2468, -5.9141) -> (-81.7017, -10.6694)
  line L17 (-87.051, -7.1502) -> (-83.2468, -5.9141)
  line L18 (-84.0377, -16.4243) -> (-87.051, -7.1502)
  line L19 (-33.7005, -80.5809) -> (-41.5895, -74.8492)
  line L20 (-31.3494, -77.3449) -> (-33.7005, -80.5809)
  line L21 (-35.3944, -74.4059) -> (-31.3494, -77.3449)
  line L22 (-22.0186, -55.9957) -> (-35.3944, -74.4059)
  line L23 (-19.6811, -47.5043) -> (-22.0186, -55.9957)
  line L24 (-39.0975, -33.3974) -> (-19.6811, -47.5043)
  line L25 (-46.4509, -38.2446) -> (-39.0975, -33.3974)
  line L26 (-59.8268, -56.6548) -> (-46.4509, -38.2446)
  line L27 (-63.8718, -53.7159) -> (-59.8268, -56.6548)
  line L28 (-66.223, -56.952) -> (-63.8718, -53.7159)
  line L29 (-58.334, -62.6837) -> (-66.223, -56.952)
  line L30 (-20.1, 81) -> (-20.1, 85)
  line L31 (-15.1, 81) -> (-20.1, 81)
  line L32 (-15.1, 58.2437) -> (-15.1, 81)
  line L33 (-12, 50) -> (-15.1, 58.2437)
  line L34 (12, 50) -> (-12, 50)
  line L35 (15.1, 58.2437) -> (12, 50)
  line L36 (15.1, 81) -> (15.1, 58.2437)
  line L37 (20.1, 81) -> (15.1, 81)
  line L38 (20.1, 85) -> (20.1, 81)
  line L39 (10.3486, 85) -> (20.1, 85)
  line L40 (-63.8718, 53.7159) -> (-66.223, 56.952)
  line L41 (-59.8268, 56.6548) -> (-63.8718, 53.7159)
  line L42 (-46.4509, 38.2446) -> (-59.8268, 56.6548)
  line L43 (-39.0975, 33.3974) -> (-46.4509, 38.2446)
  line L44 (-19.6811, 47.5043) -> (-39.0975, 33.3974)
  line L45 (-22.0186, 55.9957) -> (-19.6811, 47.5043)
  line L46 (-35.3944, 74.4059) -> (-22.0186, 55.9957)
  line L47 (-31.3494, 77.3449) -> (-35.3944, 74.4059)
  line L48 (-33.7005, 80.5809) -> (-31.3494, 77.3449)
  line L49 (-41.5895, 74.8492) -> (-33.7005, 80.5809)
  line L50 (70.8243, 44.1466) -> (74.6286, 45.3827)
  line L51 (72.3694, 39.3913) -> (70.8243, 44.1466)
  line L52 (50.7269, 32.3592) -> (72.3694, 39.3913)
  line L53 (43.8446, 26.8635) -> (50.7269, 32.3592)
  line L54 (51.261, 4.0382) -> (43.8446, 26.8635)
  line L55 (60.0592, 3.6373) -> (51.261, 4.0382)
  line L56 (81.7017, 10.6694) -> (60.0592, 3.6373)
  line L57 (83.2468, 5.9141) -> (81.7017, 10.6694)
  line L58 (87.051, 7.1502) -> (83.2468, 5.9141)
  line L59 (84.0377, 16.4243) -> (87.051, 7.1502)
  line L60 (83.2468, -5.9141) -> (87.051, -7.1502)
  line L61 (81.7017, -10.6694) -> (83.2468, -5.9141)
  line L62 (60.0592, -3.6373) -> (81.7017, -10.6694)
  line L63 (51.261, -4.0382) -> (60.0592, -3.6373)
  line L64 (43.8446, -26.8635) -> (51.261, -4.0382)
  line L65 (50.7269, -32.3592) -> (43.8446, -26.8635)
  line L66 (72.3694, -39.3913) -> (50.7269, -32.3592)
  line L67 (70.8243, -44.1466) -> (72.3694, -39.3913)
  line L68 (74.6286, -45.3827) -> (70.8243, -44.1466)
  line L69 (77.6419, -36.1086) -> (74.6286, -45.3827)
  line L70 (31.3494, 77.3449) -> (33.7005, 80.5809)
  line L71 (35.3944, 74.4059) -> (31.3494, 77.3449)
  line L72 (22.0186, 55.9957) -> (35.3944, 74.4059)
  line L73 (19.6811, 47.5043) -> (22.0186, 55.9957)
  line L74 (39.0975, 33.3974) -> (19.6811, 47.5043)
  line L75 (46.4509, 38.2446) -> (39.0975, 33.3974)
  line L76 (59.8268, 56.6548) -> (46.4509, 38.2446)
  line L77 (63.8718, 53.7159) -> (59.8268, 56.6548)
  line L78 (66.223, 56.952) -> (63.8718, 53.7159)
  line L79 (58.334, 62.6837) -> (66.223, 56.952)
  line L80 (20.1, -81) -> (20.1, -85)
  line L81 (15.1, -81) -> (20.1, -81)
  line L82 (15.1, -58.2437) -> (15.1, -81)
  line L83 (12, -50) -> (15.1, -58.2437)
  line L84 (-12, -50) -> (12, -50)
  line L85 (-15.1, -58.2437) -> (-12, -50)
  line L86 (-15.1, -81) -> (-15.1, -58.2437)
  line L87 (-20.1, -81) -> (-15.1, -81)
  line L88 (-20.1, -85) -> (-20.1, -81)
  line L89 (-10.3486, -85) -> (-20.1, -85)
  line L90 (-83.2468, 5.9141) -> (-87.051, 7.1502)
  line L91 (-81.7017, 10.6694) -> (-83.2468, 5.9141)
  line L92 (-60.0592, 3.6373) -> (-81.7017, 10.6694)
  line L93 (-51.261, 4.0382) -> (-60.0592, 3.6373)
  line L94 (-43.8446, 26.8635) -> (-51.261, 4.0382)
  line L95 (-50.7269, 32.3592) -> (-43.8446, 26.8635)
  line L96 (-72.3694, 39.3913) -> (-50.7269, 32.3592)
  line L97 (-70.8243, 44.1466) -> (-72.3694, 39.3913)
  line L98 (-74.6286, 45.3827) -> (-70.8243, 44.1466)
  line L99 (-77.6419, 36.1086) -> (-74.6286, 45.3827)
  line L100 (63.8718, -53.7159) -> (66.223, -56.952)
  line L101 (59.8268, -56.6548) -> (63.8718, -53.7159)
  line L102 (46.4509, -38.2446) -> (59.8268, -56.6548)
  line L103 (39.0975, -33.3974) -> (46.4509, -38.2446)
  line L104 (19.6811, -47.5043) -> (39.0975, -33.3974)
  line L105 (22.0186, -55.9957) -> (19.6811, -47.5043)
  line L106 (35.3944, -74.4059) -> (22.0186, -55.9957)
  line L107 (31.3494, -77.3449) -> (35.3944, -74.4059)
  line L108 (33.7005, -80.5809) -> (31.3494, -77.3449)
  line L109 (41.5895, -74.8492) -> (33.7005, -80.5809)
  circle A10 centre (0, 0) radius 4.05
  arc A11 (88.1794, -22.481) -> (89.8204, 14.6044) centre (0, 0) ccw
  arc A12 (-48.6297, -76.9166) -> (-13.8664, -89.9373) centre (0, 0) ccw
  arc A13 (-5.8682, 90.8106) -> (-41.6457, 80.9113) centre (0, 0) ccw
  arc A14 (-88.1794, 22.481) -> (-89.8204, -14.6044) centre (0, 0) ccw
  arc A15 (-58.1246, 70.0181) -> (-81.2505, 40.9799) centre (0, 0) ccw
  arc A16 (48.6297, 76.9166) -> (13.8664, 89.9373) centre (0, 0) ccw
  arc A17 (84.5526, 33.643) -> (64.082, 64.6103) centre (0, 0) ccw
  arc A18 (58.1246, -70.0181) -> (81.2505, -40.9799) centre (0, 0) ccw
  arc A19 (5.8682, -90.8106) -> (41.6457, -80.9113) centre (0, 0) ccw
  circle A20 centre (0, 0) radius 91
  line L110 (0, -91) -> (74.8212, -91)
  line L111 (74.8212, -91) -> (74.8212, -51.7956)
  constraint coincident A20 L110.start
  constraint tangent A20 L110
  constraint horizontal L110
  constraint coincident A18 L111.end
  constraint coincident A20 L111.end
  constraint vertical L111
extrude "Extrude9" [rolled back] along distance 8 taper angle 0
sketch "Sketch11" plane through (0, 0, -2) normal (0, 0, 1) x (-1, 0, 0)
  arc A0 (10.3486, 85) -> (-10.3486, 85) centre (0, 67.8855) ccw
  line L0 (10.3486, 85) -> (20.1, 85)
  line L1 (20.1, 85) -> (20.1, 81)
  line L2 (20.1, 81) -> (15.1, 81)
  line L3 (15.1, 81) -> (15.1, 58.2437)
  line L4 (15.1, 58.2437) -> (12, 50)
  line L5 (12, 50) -> (-12, 50)
  line L6 (-12, 50) -> (-15.1, 58.2437)
  line L7 (-15.1, 58.2437) -> (-15.1, 81)
  line L8 (-15.1, 81) -> (-20.1, 81)
  line L9 (-20.1, 81) -> (-20.1, 85)
  line L10 (-20.1, 85) -> (-10.3486, 85)
  circle A1 centre (0, 0) radius 26.55
  line L11 (-15.1, 79.85) -> (-21.25, 79.85)
  line L12 (-21.25, 79.85) -> (-21.25, 86.15)
  line L13 (-21.25, 86.15) -> (-14.95, 86.15)
  line L14 (-14.95, 85) -> (-14.95, 86.15)
  line L15 (-20.1, 85) -> (-14.95, 85)
  line L16 (-20.1, 85) -> (-20.1, 81)
  line L17 (-15.1, 81) -> (-20.1, 81)
  line L18 (-15.1, 81) -> (-15.1, 79.85)
  line L19 (20.1, 85) -> (14.95, 85)
  line L20 (15.1, 81) -> (20.1, 81)
  line L21 (20.1, 85) -> (20.1, 81)
  line L22 (15.1, 81) -> (15.1, 79.85)
  line L23 (15.1, 79.85) -> (21.25, 79.85)
  line L24 (21.25, 79.85) -> (21.25, 86.15)
  line L25 (14.95, 85) -> (14.95, 86.15)
  line L26 (21.25, 86.15) -> (14.95, 86.15)
  circle A2 centre (0, 0) radius 4.05
  line L27 (-74.8212, 91) -> (-74.8212, 51.7956)
  arc A3 (-74.8212, 51.7956) -> (0, 91) centre (0, 0) ccw
  line L28 (0, 91) -> (-74.8212, 91)
extrude "Extrude10" [rolled back] along distance -5 taper angle 0
extrude "Extrude11" [rolled back] along distance -40 taper angle 0
sketch "Sketch12" plane through (0, 0, 0) normal (1, 0, 0) x (0, 1, 0)
move_body "Move1" [rolled back]
pasted_body "CopyPasteBodies1" makes body 4
move_body "Move2" [rolled back]
sketch "Sketch14" plane through (0, 0, 0) normal (1, 0, 0) x (0, 1, 0)
  circle A0 centre (-60.35, -13.5) radius 18.5
  circle A1 centre (-60.35, -13.5) radius 15.5
  line L0 (-60.35, -13.5) -> (-67.6967, -30.4787)
  line L1 (-60.35, -13.5) -> (-60.8671, 4.9928)
  line L2 (-79.85, -10) -> (-79.85, -42)
  circle A2 centre (-60.35, -13.5) radius 20.5
  line L3 (-79.85, -42) -> (-79.85, 8.316)
  line L4 (-81, -2) -> (-58.2437, -2)
  line L5 (-103, -8) -> (-66, -8) construction
  circle A3 centre (-90.9861, -8) radius 11.65
  line L6 (-81.0625, -1.8973) -> (-85.0624, -1.8842)
  arc A4 (-85.0624, -1.8842) -> (-90.9861, -8) centre (-85.0817, -7.7923) ccw
  circle A5 centre (-90.9861, -8) radius 1.5
  line L7 (-86.15, -10) -> (-86.15, -42)
  line L8 (-86.15, -22.9599) -> (-86.15, 5)
  arc A6 (-86.15, -5.3805) -> (-86.15, -10.6195) centre (-90.9861, -8) ccw
  dimension "d65" = 37
  dimension "d66" = 3
  dimension "d73" = 155
  dimension "d80" = 2
  dimension "d81" = 19.5
  dimension "d179" = 11.5
  dimension "d188" = 6
  dimension "d189" = 23.3
  dimension "d190" = 4
  dimension "d191" = 11
  dimension "d192" = 3
  constraint concentric A0 A1
  constraint coincident A0.centre A1.centre
  constraint coincident A0 L0.end
  constraint coincident A0 L1.end
  constraint concentric A0 A2
  constraint coincident L2.end L3.start
  constraint horizontal L5
  constraint coincident L5 A3.centre
  constraint coincident L4.start A3
  constraint coincident A3.centre A4.end
  constraint tangent L6 A4
  constraint coincident A3 L6.start
  constraint concentric A3 A6
  constraint concentric A3 A5
  constraint coincident L7 L8.start
  constraint vertical L8
  constraint coincident L8 A6.start
  constraint coincident L7 A6.end
  measures "d65" diameter of A0
  measures "d66" distance of A0 A1
  measures "d73" angle of L0 L1
  measures "d80" distance of A0 A2
  measures "d81" distance of A0.centre L3
  measures "d179" distance of A0.centre L4
  measures "d188" distance of L4 L5
  measures "d189" diameter of A3
  measures "d190" distance of L6.start L6.end
  measures "d191" diameter of A6
  measures "d192" diameter of A5
move_body "Move3" [rolled back]
sketch "Sketch16" plane through (0, 0, -10) normal (0, 0, -1) x (1, 0, 0)
  line L0 (21.25, 79.85) -> (15.1, 79.85)
  line L1 (15.1, 79.85) -> (15.1, 58.2437)
  line L2 (15.1, 58.2437) -> (12, 50)
  line L3 (12, 50) -> (-12, 50)
  line L4 (-12, 50) -> (-15.1, 58.2437)
  line L5 (-15.1, 58.2437) -> (-15.1, 79.85)
  line L6 (-15.1, 79.85) -> (-21.25, 79.85)
  line L7 (-21.25, 79.85) -> (-21.25, 86.15)
  line L8 (-21.25, 86.15) -> (-14.95, 86.15)
  arc A0 (10.3486, 85) -> (-10.3486, 85) centre (0, 67.8855) ccw
  line L9 (10.3486, 85) -> (14.95, 85)
  line L10 (14.95, 85) -> (14.95, 86.15)
  line L11 (14.95, 86.15) -> (21.25, 86.15)
  line L12 (21.25, 86.15) -> (21.25, 79.85)
  circle A1 centre (0, 0) radius 31
  circle A2 centre (0, 0) radius 11.15
  line L13 (-14.95, 86.15) -> (-14.95, 85)
  line L14 (-14.95, 85) -> (-10.3486, 85)
  circle A3 centre (0, 0) radius 4.05
  line L15 (74.8212, 51.7956) -> (74.8212, 91)
  line L16 (74.8212, 91) -> (0, 91)
  arc A4 (0, 91) -> (74.8212, 51.7956) centre (0, 0) ccw
  dimension "d82" = 62
  dimension "d83" = 22.3
  constraint concentric A1 A2
  measures "d82" diameter of A1
  measures "d83" diameter of A2
extrude "Extrude12" [rolled back] along distance 6 taper angle 0
extrude "Extrude13" [rolled back] along distance 3 taper angle 0
extrude "Extrude14" [rolled back] along distance 19 taper angle 0
pattern_circular "C-Pattern2" [rolled back] count u 10 total angle 360
extrude "Extrude15" [rolled back] along distance 15 taper angle 0
sketch "Sketch18" plane through (15, 0, 0) normal (1, 0, 0) x (0, 1, 0)
  arc A0 (-67.6967, -30.4787) -> (-60.8671, 4.9928) centre (-60.35, -13.5) ccw
  line L0 (-60.8671, 4.9928) -> (-60.7833, 1.9939)
  arc A1 (-66.5054, -27.7254) -> (-60.7833, 1.9939) centre (-60.35, -13.5) ccw
  line L1 (-66.5054, -27.7254) -> (-67.6967, -30.4787)
  line L2 (-60.35, -13.5) -> (-60.8671, 4.9928)
  line L3 (-60.35, -13.5) -> (-67.6967, -30.4787)
  circle A2 centre (-60.35, -13.5) radius 18.5
  circle A3 centre (-60.35, -13.5) radius 10
  circle A4 centre (-60.35, -13.5) radius 3.925
  circle A5 centre (-59.3239, 3.469) radius 1.5
  dimension "d98" = 20
  dimension "d103" = 7.85
  constraint coincident A0.centre A1.centre
  constraint tangent L0 A5
  constraint tangent A0 A5
  constraint tangent A1 A5
  measures "d98" diameter of A3
  measures "d103" diameter of A4
extrude "Extrude16" [rolled back] along distance 3 taper angle 0